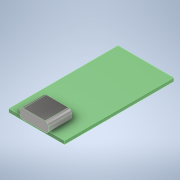
# Autodesk Inventor part: MCU_TinyPICO
Saved by Autodesk Inventor 2022 (Build 260153000, 153)
## iProperties
Created: 2022-12-31
Part Number: MCU_TinyPICO
Material: Generic
Document SubType Name: Modeling
Designer: karpova
Density: 1 g/cm^3
Appearance: Smooth - Dark Forest Green
Author: karpova
Autodesk Inventor part; units mm, degrees
ref_plane "YZ Plane" through (0, 0, 0) normal (1, 0, 0) x (0, 1, 0)
ref_plane "XZ Plane" through (0, 0, 0) normal (0, 1, 0) x (-1, 0, 0)
sketch "Sketch1" plane through (0, 0, 0) normal (0, 1, 0) x (-1, 0, 0)
  line L0 (0, 0) -> (34.5, 0)
  line L1 (34.5, 0) -> (34.5, -17.6)
  line L2 (34.5, -17.6) -> (0, -17.6)
  line L3 (0, -17.6) -> (0, 0)
  dimension "d0" = 17.6
  dimension "d1" = 34.5
  constraints: 8 end point, 2 parallel, 1 horizontal, 1 perpendicular
  measures "d0" distance of L0.end L1.end
  measures "d1" distance of L1.end L2.end
extrude "Extrusion1" add sketch "Sketch1" along normal blind 1.05
ref_plane "Work Plane1" through (0.8, 0, 0) normal (1, 0, 0) x (0, 0, -1)
sketch "Sketch2" plane through (0.8, 0, 0) normal (1, 0, 0) x (0, 0, -1)
  line L0 (0, 0) -> (17.6, 0) projected
  line L1 (17.6, 0) -> (17.6, 1.05) projected
  line L2 (0, 1.05) -> (17.6, 1.05) projected
  line L3 (0, 0) -> (0, 1.05) projected
  line L4 (17.6, 0) -> (0, 0) construction
  line L5 (8.8, 0) -> (8.8, 1.05) construction
  line L6 (17.6, 1.05) -> (0, 1.05) construction
  line L7 (5.34, 4.22) -> (12.26, 4.22)
  line L8 (13.3, 3.18) -> (13.3, 2.09)
  line L9 (12.26, 1.05) -> (5.34, 1.05)
  line L10 (4.3, 2.09) -> (4.3, 3.18)
  line L11 (0, 1.05) -> (17.6, 1.05) projected
  arc A0 (5.34, 4.22) -> (4.3, 3.18) centre (5.34, 3.18) ccw
  arc A1 (4.3, 2.09) -> (5.34, 1.05) centre (5.34, 2.09) ccw
  arc A2 (13.3, 3.18) -> (12.26, 4.22) centre (12.26, 3.18) ccw
  arc A3 (12.26, 1.05) -> (13.3, 2.09) centre (12.26, 2.09) ccw
  point P0 (4.3, 4.22)
  point P1 (13.3, 4.22)
  point P2 (4.3, 1.05)
  point P3 (5.34, 1.05)
  point P4 (12.26, 1.05)
  dimension "d5" = 9
  dimension "d6" = 3.17
  dimension "d7" = 1.04
  constraints: 10 end point, 8 point on circle, 8 tangent, 6 point on line, 4 centre point, 3 equal radius, 2 midpoint, 2 parallel, 1 collinear, 1 horizontal, 1 perpendicular, 1 other
  measures "d5" distance of point (4.3, 4.22) point (13.3, 4.22)
  measures "d6" distance of point (4.3, 1.05) point (4.3, 4.22)
  measures "d7" radius of A0
extrude "Extrusion2" add sketch "Sketch2" against normal blind 7.35 contours A1 L10 A0 L7 A2 L8 A3 L2
equation "\"d2\" = pcbThickness"
equation "\"pcbThickness\" = 1.05"
equation "\"usbcEdgeOffset\" = 0.8"
equation "\"d4\" = usbcEdgeOffset"
body "Solid1"
